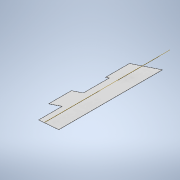
# Autodesk Inventor part: mainPartHouseRoof
Saved by Autodesk Inventor 2022.1 (Build 261234000, 234)
## iProperties
Created: 2021-07-13
Part Number: mainPartHouseRoof
Material: Generic
Document SubType Name: Modeling
Designer: robst
Density: 1 g/cm^3
Appearance: Default
Author: robst
Autodesk Inventor part; units mm, degrees
ref_plane "YZ Plane" through (0, 0, 0) normal (1, 0, 0) x (0, 1, 0)
ref_plane "Work Plane3" through (0, 0, 0) normal (-0.7071068, 0.7071068, 0) x (0, 0, 1)
sketch "Sketch9" plane through (0, 0, 0) normal (-0.7071068, 0.7071068, 0) x (0, 0, 1)
  line L0 (0, 0) -> (0, -3810)
  line L1 (0, -3810) -> (3987.8, -3810)
  line L2 (3987.8, -3810) -> (3987.8, 0)
  line L3 (0, 0) -> (3987.8, 0)
  line L4 (3987.8, -3810) -> (9652, -3810) construction
  line L5 (9652, -3810) -> (9652, 0)
  line L6 (9652, 0) -> (16510, 0)
  line L7 (15697.2, -3810) -> (9652, -3810)
  line L8 (15697.2, -3810) -> (16510, 0)
  dimension "d39" = 3810
  dimension "d40" = 3987.8
  dimension "d53" = 5664.2
  dimension "d54" = 6045.2
  dimension "d55" = 6858
  constraints: 18 end point, 3 horizontal, 2 perpendicular, 2 vertical
  measures "d39" distance of L0.start L0.end
  measures "d40" distance of L0.end L1.end
  measures "d53" distance of L1.end L4.end
  measures "d54" distance of L7.start L4.end
  measures "d55" distance of L5.end L6.end
ref_plane "4-12pictchWorkPlane" through (-2694.0768, -2694.0768, 0) normal (-0.3162286, 0.948683, 0) x (0, 0, 1)
sketch "Sketch10" plane through (-2694.0768, -2694.0768, 0) normal (-0.3162286, 0.948683, 0) x (0, 0, 1)
  line L0 (0, 0) -> (0, -2184.4)
  line L1 (0, -2184.4) -> (3860.8, -2184.4)
  line L2 (3860.8, -2184.4) -> (3860.8, -1549.4)
  line L3 (3860.8, -1549.4) -> (8026.4, -1549.4)
  line L4 (8026.4, -1549.4) -> (8026.4, -3581.4)
  line L5 (8026.4, -3581.4) -> (11684, -3581.4)
  line L6 (11684, -3581.4) -> (11684, -1295.4)
  line L7 (11684, -1295.4) -> (15468.6, -1295.4)
  line L8 (15468.6, -1295.4) -> (15468.6, 3407.7691) construction
  line L9 (17156.3434, 3407.7691) -> (0, 3407.7691)
  line L10 (15468.6, 3407.7691) -> (16687.8, 3407.7691) construction
  line L11 (15468.6, -1295.4) -> (16687.8, 3407.7691)
  line L12 (0, 0) -> (15804.4058, 0)
  line L13 (0, 0) -> (0, 3407.7691)
  line L14 (0, 3407.7691) -> (16687.8, 3407.7691)
  dimension "d42" = 2184.4
  dimension "d43" = 3860.8
  dimension "d44" = 635
  dimension "d45" = 4165.6
  dimension "d46" = 2032
  dimension "d47" = 3657.6
  dimension "d48" = 2286
  dimension "d49" = 3784.6
  dimension "d50" = 1219.2
  dimension "d58" = 90
  constraints: 30 end point, 6 perpendicular, 3 horizontal, 3 vertical, 2 point on line, 1 collinear
  measures "d42" distance of L0.start L0.end
  measures "d43" distance of L0.end L1.end
  measures "d44" distance of L1.end L2.end
  measures "d45" distance of L2.end L3.end
  measures "d46" distance of L3.end L4.end
  measures "d47" distance of L4.end L5.end
  measures "d48" distance of L5.end L6.end
  measures "d49" distance of L6.end L7.end
  measures "d50" distance of L8.end L10.end
  measures "d58" angle of L8 L10
extrude "Extrusion8" add sketch "Sketch10" against normal blind 25.4
extrude "Extrusion9" add sketch "Sketch9" against normal blind 25.4
equation "\"pitch_4_12\" = 18.435deg"
equation "\"pitch_12_12\" = 45deg"
equation "\"d41\" = pitch_4_12"
body "Solid2"
